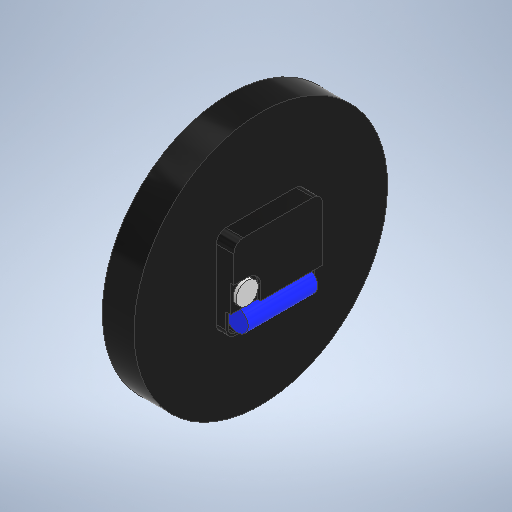
# Autodesk Inventor part: Clack
Saved by Autodesk Inventor 2025.2 (Build 292293000, 293)
## iProperties
Created: 2026-02-21
Part Number: Clack
Material: 一般
Document SubType Name: Modeling
Designer: naka6
Density: 1 g/cm^3
Appearance: 既定
Author: naka6
Autodesk Inventor part; units mm, degrees
ref_plane "YZ Plane" through (0, 0, 0) normal (1, 0, 0) x (0, 1, 0)
ref_plane "XZ Plane" through (0, 0, 0) normal (0, 1, 0) x (-1, 0, 0)
ref_plane "XY Plane" through (0, 0, 0) normal (0, 0, 1) x (1, 0, 0)
sketch "スケッチ1" plane through (0, 0, 0) normal (1, 0, 0) x (0, 1, 0)
  circle A0 centre (0, 0) radius 80
  dimension "d0" = 160
  constraints: 1 centre point, 1 coincident
  measures "d0" diameter of A0
extrude "押し出し1" add sketch "スケッチ1" along normal blind 20
sketch "スケッチ2" plane through (20, 0, 0) normal (1, 0, 0) x (0, 0, -1)
  line L0 (28, -28) -> (-28, -28)
  line L1 (-28, -28) -> (-28, 28)
  line L2 (-28, 28) -> (28, 28)
  line L3 (28, 28) -> (28, -28)
  line L4 (28, -28) -> (-28, 28) construction
  line L5 (-28, -28) -> (28, 28) construction
  point P0 (0, 0)
  dimension "d3" = 56
  dimension "d4" = 56
  constraints: 12 end point, 2 midpoint, 2 parallel, 1 horizontal, 1 perpendicular
  measures "d3" distance of L1.end L2.end
  measures "d4" distance between parallel lines of L0 L2
extrude "押し出し2" add sketch "スケッチ2" along normal blind 11
sketch "スケッチ3" plane through (31, 0, 0) normal (1, 0, 0) x (0, 0, -1)
  line L0 (28, 28) -> (-28, 28) projected
  line L1 (-28, 28) -> (-28, -28) projected
  line L2 (-28, -28) -> (28, -28) projected
  line L3 (28, -28) -> (28, 28) projected
  circle A0 centre (-22, 22) radius 6
  line L4 (0, 28) -> (0, -28)
  line L5 (-28, 0) -> (28, 0)
  circle A1 centre (22, 22) radius 6
  circle A2 centre (-22, -22) radius 6
  circle A3 centre (22, -22) radius 6
  point P0 (0, 0)
  point P1 (-22, -28)
  point P2 (-28, -22)
  point P3 (28, -22)
  point P4 (22, -28)
  point P5 (22, 28)
  point P6 (28, 22)
  point P7 (-28, 22)
  point P8 (-22, 28)
  dimension "d7" = 12
  constraints: 4 centre point, 4 end point, 4 midpoint, 3 symmetric about line, 2 tangent, 3 other
  measures "d7" diameter of A0
extrude "押し出し3" cut sketch "スケッチ3" against normal up to surface (11 mm away) contours L3 A1 L0 | A0 L1 L0 | L3 L2 A3 | L2 L1 A2
sketch "スケッチ4" plane through (31, 0, 0) normal (1, 0, 0) x (0, 0, -1)
  arc A0 (22, -28) -> (28, -22) centre (22, -22) ccw projected
  line L0 (28, -22) -> (28, 22) projected
  arc A1 (28, 22) -> (22, 28) centre (22, 22) ccw projected
  line L1 (22, 28) -> (-22, 28) projected
  arc A2 (-22, 28) -> (-28, 22) centre (-22, 22) ccw projected
  line L2 (-28, 22) -> (-28, -22) projected
  arc A3 (-28, -22) -> (-22, -28) centre (-22, -22) ccw projected
  line L3 (-22, -28) -> (22, -28) projected
  line L4 (-28, -12) -> (28, -12)
  point P0 (0, 0)
  dimension "d10" = 16
  constraints: 2 end point, 2 point on line, 1 perpendicular
  measures "d10" distance between parallel lines of L3 L4
extrude "押し出し4" cut sketch "スケッチ4" against normal blind 5 contours L3 A3 L2 L4 L0 A0
sketch "スケッチ5" plane through (26, 0, 0) normal (1, 0, 0) x (0, 0, -1)
  line L0 (28, -12) -> (28, -22) projected
  line L1 (-28, -12) -> (28, -12) projected
  line L2 (-28, -22) -> (-28, -12) projected
  arc A0 (-28, -22) -> (-22, -28) centre (-22, -22) ccw projected
  line L3 (22, -28) -> (-22, -28) projected
  arc A1 (22, -28) -> (28, -22) centre (22, -22) ccw projected
  arc A2 (-26.5, -22) -> (-22, -26.5) centre (-22, -22) ccw
  line L4 (-26.5, -22) -> (-26.5, -13.5)
  line L5 (-26.5, -13.5) -> (26.5, -13.5)
  line L6 (26.5, -13.5) -> (26.5, -22)
  arc A3 (22, -26.5) -> (26.5, -22) centre (22, -22) ccw
  line L7 (22, -26.5) -> (-22, -26.5)
  line L8 (-26.5, -13.5) -> (-26.5, -12)
  line L9 (26.5, -13.5) -> (26.5, -12)
  point P0 (0, 0)
  dimension "d13" = 1.5
  constraints: 12 end point, 4 point on circle, 2 centre point, 2 perpendicular, 2 point on line, 5 other
  measures "d13" radial gap between concentric circles of A0 A2
extrude "押し出し5" cut sketch "スケッチ5" against normal up to surface (6 mm away) contours L9 L5 L8 L1 | L6 A3 L7 A2 L4 L5
ref_plane "作業平面1" through (26, -22, -22.1) normal (0, 0, 1) x (1, 0, 0)
sketch "スケッチ6" plane through (26, -22, -22.1) normal (0, 0, 1) x (1, 0, 0)
  line L0 (0, 10) -> (-6, 10) projected
  line L1 (0, 10) -> (5, 10) projected
  line L2 (-6, -58) -> (-6, 102) projected
  circle A0 centre (1, 3) radius 7
  point P0 (-26, 22)
  dimension "d17" = 14
  constraints: 2 tangent, 1 centre point
  measures "d17" diameter of A0
extrude "押し出し6" add sketch "スケッチ6" along normal blind 44 contours A0
sketch "スケッチ7" plane through (31, 0, 0) normal (1, 0, 0) x (0, 0, -1)
  line L0 (-28, -12) -> (28, -12) projected
  line L1 (28, -12) -> (28, 22) projected
  arc A0 (28, 22) -> (22, 28) centre (22, 22) ccw projected
  line L2 (22, 28) -> (-22, 28) projected
  arc A1 (-22, 28) -> (-28, 22) centre (-22, 22) ccw projected
  line L3 (-28, 22) -> (-28, -12) projected
  line L4 (-28, -12) -> (-11, -12)
  line L5 (-11, -12) -> (-11, 5)
  line L6 (-11, 5) -> (-28, 5)
  line L7 (-28, 5) -> (-28, -12)
  circle A2 centre (-19, -3) radius 8
  point P0 (0, 0)
  point P1 (-19, 5)
  point P2 (-11, -3)
  dimension "d20" = 17
  dimension "d21" = 17
  dimension "d22" = 16
  constraints: 8 end point, 2 parallel, 2 tangent, 1 centre point, 1 horizontal, 1 perpendicular
  measures "d20" distance of L6.end L5.end
  measures "d21" distance of L4.end L5.end
  measures "d22" diameter of A2
extrude "押し出し7" cut sketch "スケッチ7" against normal blind 2 contours L3 L6 A2 L5 L0 | A2
sketch "スケッチ8" plane through (29, 0, 0) normal (1, 0, 0) x (0, 0, -1)
  line L0 (-28, -12) -> (-28, 5) projected
  line L1 (-11, -12) -> (-28, -12) projected
  line L2 (-11, -3) -> (-11, -12) projected
  arc A0 (-11, -3) -> (-19, 5) centre (-19, -3) ccw projected
  line L3 (-28, 5) -> (-19, 5) projected
  circle A1 centre (-19.5, -3.5) radius 7
  point P0 (0, 0)
  dimension "d25" = 14
  dimension "d26" = 8.5
  dimension "d27" = 8.5
  constraints: 1 centre point
  measures "d25" diameter of A1
  measures "d26" distance from line of L0 A1.centre
  measures "d27" distance from line of L1 A1.centre
extrude "押し出し8" add sketch "スケッチ8" along normal blind 2 contours A1
